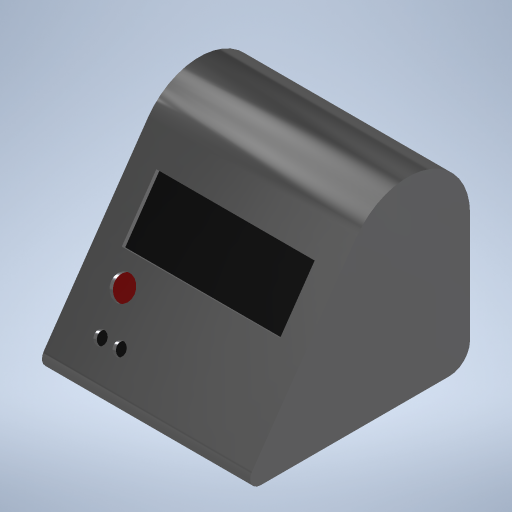
# Autodesk Inventor part: caja del arduino
Saved by Autodesk Inventor 2023 (Build 270158000, 158)
## iProperties
Created: 2022-10-13
Part Number: caja del arduino
Material: Generic
Document SubType Name: Modeling
Designer: Xiaba
Density: 1 g/cm^3
Appearance: Default
Author: Xiaba
Autodesk Inventor part; units mm, degrees
ref_plane "YZ Plane" through (0, 0, 0) normal (1, 0, 0) x (0, 1, 0)
ref_plane "XZ Plane" through (0, 0, 0) normal (0, 1, 0) x (-1, 0, 0)
ref_plane "XY Plane" through (0, 0, 0) normal (0, 0, 1) x (1, 0, 0)
sketch "Sketch1" plane through (0, 0, 0) normal (1, 0, 0) x (0, 1, 0)
  circle A0 centre (6.2867, -6.541) radius 3
  line L0 (6.2867, -9.541) -> (1, -9.541)
  line L1 (0, -8.541) -> (0, 0.5151)
  line L2 (0.785, 0.926) -> (7.9965, -4.0759)
  arc A1 (0.785, 0.926) -> (0, 0.5151) centre (0.5, 0.5151) ccw
  arc A2 (0, -8.541) -> (1, -9.541) centre (1, -8.541) ccw
  point P0 (0, 0)
  dimension "d0" = 6
  dimension "d1" = 0.5
  dimension "d2" = 1
  constraints: 6 end point, 6 point on circle, 6 tangent, 3 centre point, 1 horizontal, 1 perpendicular
  measures "d0" diameter of A0
  measures "d1" radius of A1
  measures "d2" radius of A2
extrude "Extrusion1" add sketch "Sketch1" along normal blind 10
shell "Shell1" thickness 0.5 removed faces 0
sketch "Sketch2" plane through (0, 0.785, 0.926) normal (0, 0.5699242, 0.8216972) x (1, 0, 0)
  line L0 (0, 8.7764) -> (0, 0) projected
  line L1 (0, 0) -> (10, 0) projected
  line L2 (10, 8.7764) -> (10, 0) projected
  line L3 (0, 8.7764) -> (10, 8.7764) projected
  line L4 (1.2, 7.3764) -> (8.8, 7.3764)
  line L5 (8.8, 7.3764) -> (8.8, 4.4678)
  line L6 (8.8, 4.4678) -> (1.2, 4.4678)
  line L7 (1.2, 4.4678) -> (1.2, 7.3764)
  circle A0 centre (1.94, 3.259) radius 0.5615
  circle A1 centre (1.94, 1.3767) radius 0.3
  circle A2 centre (2.8563, 1.3767) radius 0.3
  point P0 (0, -0.1173)
  dimension "d6" = 1.4
  dimension "d7" = 1.2
  dimension "d8" = 1.2
  dimension "d9" = 0.6
  dimension "d10" = 0.6
  constraints: 8 end point, 3 centre point, 2 parallel, 1 horizontal, 1 perpendicular
  measures "d6" distance between parallel lines of L4 L3
  measures "d7" distance between parallel lines of L5 L2
  measures "d8" distance between parallel lines of L0 L7
  measures "d9" diameter of A1
  measures "d10" diameter of A2
extrude "Extrusion2" cut sketch "Sketch2" against normal blind 0.2 contours L4 L5 L6 L7 | A0 | A1 | A2
sketch "Sketch3" plane through (0, 1, -9.541) normal (0, 0, -1) x (-1, 0, 0)
  circle A0 centre (-5, 2.6434) radius 0.7
  line L0 (0, 0) -> (0, 5.2867) projected
  line L1 (0, 5.2867) -> (-10, 5.2867) projected
  line L2 (-10, 0) -> (-10, 5.2867) projected
  line L3 (0, 0) -> (-10, 0) projected
  point P0 (0, -1)
  dimension "d13" = 1.4
  constraints: 1 centre point
  measures "d13" diameter of A0
extrude "Extrusion3" cut sketch "Sketch3" against normal blind 1 contours A0
body "Solid1"
